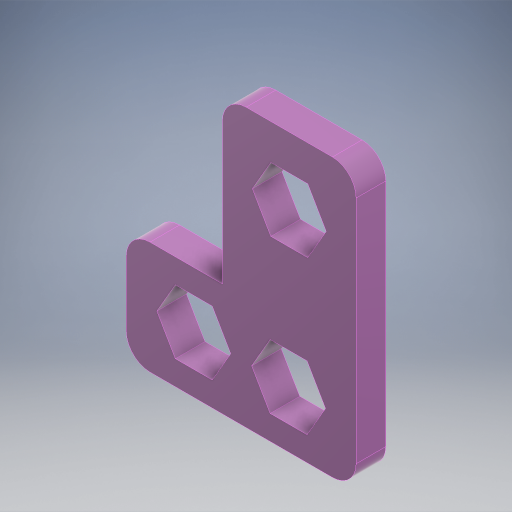
# Autodesk Inventor part: М3x3 вставка
Saved by Autodesk Inventor 2023 (Build 270158000, 158)
## iProperties
Created: 2023-03-26
Part Number: М3x3 вставка
Material: Типовые
Document SubType Name: Modeling
Designer: Admin
Density: 1 g/cm^3
Appearance: По умолчанию
Author: Admin
Autodesk Inventor part; units mm, degrees
ref_plane "YZ Plane" through (0, 0, 0) normal (1, 0, 0) x (0, 1, 0)
ref_plane "XZ Plane" through (0, 0, 0) normal (0, 1, 0) x (-1, 0, 0)
ref_plane "XY Plane" through (0, 0, 0) normal (0, 0, 1) x (1, 0, 0)
sketch "Эскиз1" plane through (0, 0, 0) normal (0, 0, 1) x (1, 0, 0)
  arc A0 (-11.7585, -8.22) -> (-13.7585, -10.22) centre (-11.7585, -10.22) ccw
  arc A1 (3.6415, -17.72) -> (5.6415, -15.72) centre (3.6415, -15.72) ccw
  line L0 (5.6415, -15.72) -> (5.6415, -10.22)
  arc A2 (5.6415, -10.22) -> (3.6415, -8.22) centre (3.6415, -10.22) ccw
  line L1 (3.6415, -8.22) -> (-11.7585, -8.22)
  line L2 (-11.7585, -17.72) -> (3.6415, -17.72)
  arc A3 (-13.7585, -15.72) -> (-11.7585, -17.72) centre (-11.7585, -15.72) ccw
  line L3 (-13.7585, -10.22) -> (-13.7585, -15.72)
  line L4 (-1.5588, 2.7) -> (1.5588, 2.7)
  line L5 (1.5588, 2.7) -> (3.1177, 0)
  line L6 (3.1177, 0) -> (1.5588, -2.7)
  line L7 (1.5588, -2.7) -> (-1.5588, -2.7)
  line L8 (-1.5588, -2.7) -> (-3.1177, 0)
  line L9 (-3.1177, 0) -> (-1.5588, 2.7)
  circle A4 centre (0, 0) radius 1.5
  line L10 (5.6415, 3.7) -> (5.6415, -10.22)
  line L11 (-5.6415, 3.7) -> (-5.6415, -8.22)
  line L12 (-3.6415, 5.7) -> (3.6415, 5.7)
  arc A5 (-3.6415, 5.7) -> (-5.6415, 3.7) centre (-3.6415, 3.7) ccw
  arc A6 (5.6415, 3.7) -> (3.6415, 5.7) centre (3.6415, 3.7) ccw
  circle A7 centre (-8.0585, -12.97) radius 1.5
  circle A8 centre (-0.0585, -12.97) radius 1.5
  line L13 (-9.6173, -10.27) -> (-6.4997, -10.27)
  line L14 (-6.4997, -10.27) -> (-4.9408, -12.97)
  line L15 (-4.9408, -12.97) -> (-6.4997, -15.67)
  line L16 (-6.4997, -15.67) -> (-9.6173, -15.67)
  line L17 (-9.6173, -15.67) -> (-11.1762, -12.97)
  line L18 (-11.1762, -12.97) -> (-9.6173, -10.27)
  line L19 (-1.6173, -10.27) -> (1.5003, -10.27)
  line L20 (1.5003, -10.27) -> (3.0592, -12.97)
  line L21 (3.0592, -12.97) -> (1.5003, -15.67)
  line L22 (1.5003, -15.67) -> (-1.6173, -15.67)
  line L23 (-1.6173, -15.67) -> (-3.1762, -12.97)
  line L24 (-3.1762, -12.97) -> (-1.6173, -10.27)
  line L25 (-4.0585, -8.22) -> (-4.0585, -7.9956) construction
  point P0 (0, 0)
  point P1 (37.3067, 7.3314)
  point P2 (0, 0)
  point P3 (0, 0)
  point P4 (5.6415, -12.97)
  point P5 (-13.7585, -12.97)
  point P6 (-5.258, -5.555)
  point P7 (0, 5.7)
  dimension "d33" = 3
  dimension "d34" = 2
  dimension "d39" = 4.2
  dimension "d41" = 3
  dimension "d43" = 11.283
  constraints: 50 end point, 12 point on circle, 10 tangent, 9 centre point, 7 equal radius, 6 parallel, 5 coincident, 4 horizontal, 3 horizontal alignment, 3 midpoint, 3 vertical, 2 equal length, 1 perpendicular, 1 point on line, 1 vertical alignment, 46 other
  measures "d33" diameter of A4
  measures "d34" radius of A6
  measures "d39" distance edge to line of A7 L3
  measures "d41" distance between parallel lines of L12 L4
  measures "d43" distance between parallel lines of L11 L10
extrude "Выдавливание1" add sketch "Эскиз1" along normal blind 2.5 contours L1 A2 L0 A1 L2 A3 L3 A0 | L11 A5 L12 A6 L10 A2 L1
